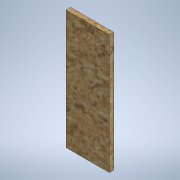
# Autodesk Inventor part: зад
Saved by Autodesk Inventor 2022 (Build 260153000, 153)
## iProperties
Created: 2021-10-11
Part Number: зад
Material: Типовые
Document SubType Name: Modeling
Designer: Admin
Density: 1 g/cm^3
Appearance: Древесно-стружечная плита
Author: Admin
Autodesk Inventor part; units mm, degrees
ref_plane "YZ Plane" through (0, 0, 0) normal (1, 0, 0) x (0, 1, 0)
ref_plane "XZ Plane" through (0, 0, 0) normal (0, 1, 0) x (-1, 0, 0)
ref_plane "XY Plane" through (0, 0, 0) normal (0, 0, 1) x (1, 0, 0)
sketch "Эскиз1" plane through (0, 0, 0) normal (0, 0, 1) x (1, 0, 0)
  line L0 (-72.5, -200) -> (72.5, -200)
  line L1 (72.5, -200) -> (72.5, 200)
  line L2 (72.5, 200) -> (-72.5, 200)
  line L3 (-72.5, 200) -> (-72.5, -200)
  line L4 (-72.5, -200) -> (72.5, 200) construction
  line L5 (72.5, -200) -> (-72.5, 200) construction
  point P0 (0, 0)
  dimension "d0" = 145
  dimension "d1" = 400
  constraints: 12 end point, 2 midpoint, 2 parallel, 1 horizontal, 1 perpendicular
  measures "d0" distance of L2.end L1.end
  measures "d1" distance of L1.end L0.end
extrude "Выдавливание1" add sketch "Эскиз1" along normal blind 15
